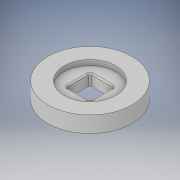
# Autodesk Inventor part: gear_collar_small
Saved by Autodesk Inventor 2019.3 (Build 233278000, 278)
## iProperties
Created: 2019-01-25
Part Number: gear_collar_small
Material: Generic
Document SubType Name: Modeling
Designer: Varga Daniel
Density: 1 g/cm^3
Appearance: Default
Author: Varga Daniel
Autodesk Inventor part; units mm, degrees
ref_plane "YZ Plane" through (0, 0, 0) normal (1, 0, 0) x (0, 1, 0)
ref_plane "XZ Plane" through (0, 0, 0) normal (0, 1, 0) x (-1, 0, 0)
ref_plane "XY Plane" through (0, 0, 0) normal (0, 0, 1) x (1, 0, 0)
derived "Base_part.ipt"
sketch "Axle_hole_sketch" plane through (0, 0, 0) normal (0, 1, 0) x (-1, 0, 0)
  line L0 (-14.3207, 2.4447) -> (-17.4707, 2.4447)
  line L1 (-17.7707, 2.7447) -> (-17.7707, 5.8947)
  line L2 (-17.4707, 6.1947) -> (-14.3207, 6.1947)
  line L3 (-14.0207, 5.8947) -> (-14.0207, 2.7447)
  line L4 (-14.0207, 2.4447) -> (-17.7707, 6.1947) construction
  line L5 (-17.7707, 2.4447) -> (-14.0207, 6.1947) construction
  arc A0 (-14.3207, 2.4447) -> (-14.0207, 2.7447) centre (-14.3207, 2.7447) ccw
  arc A1 (-17.7707, 2.7447) -> (-17.4707, 2.4447) centre (-17.4707, 2.7447) ccw
  arc A2 (-17.4707, 6.1947) -> (-17.7707, 5.8947) centre (-17.4707, 5.8947) ccw
  arc A3 (-14.0207, 5.8947) -> (-14.3207, 6.1947) centre (-14.3207, 5.8947) ccw
  point P0 (0, 0)
  point P1 (-15.8957, 4.3197)
sketch "Sketch1" plane through (0, 0, 0) normal (0, 1, 0) x (-1, 0, 0)
  circle A0 centre (0, 0) radius 6.5
  dimension "d2" = 13
  constraints: 1 centre point, 1 coincident
  measures "d2" diameter of A0
extrude "Extrusion1" add sketch "Sketch1" along normal blind 2.5
sketch "Sketch2" plane through (0, 2.5, 0) normal (0, 1, 0) x (1, 0, 0)
  line L0 (-1.575, -1.875) -> (1.575, -1.875)
  line L1 (1.875, -1.575) -> (1.875, 1.575)
  line L2 (1.575, 1.875) -> (-1.575, 1.875)
  line L3 (-1.875, 1.575) -> (-1.875, -1.575)
  line L4 (-1.875, -1.875) -> (1.875, 1.875) construction
  line L5 (1.875, -1.875) -> (-1.875, 1.875) construction
  arc A0 (-1.575, 1.875) -> (-1.875, 1.575) centre (-1.575, 1.575) ccw
  arc A1 (-1.875, -1.575) -> (-1.575, -1.875) centre (-1.575, -1.575) ccw
  arc A2 (1.575, -1.875) -> (1.875, -1.575) centre (1.575, -1.575) ccw
  arc A3 (1.875, 1.575) -> (1.575, 1.875) centre (1.575, 1.575) ccw
  line L6 (14.3207, -2.4447) -> (17.4707, -2.4447) construction
  line L7 (14.0207, -5.8947) -> (14.0207, -2.7447) construction
  arc A4 (14.3207, -2.4447) -> (14.0207, -2.7447) centre (14.3207, -2.7447) ccw construction
  line L8 (17.7707, -2.7447) -> (17.7707, -5.8947) construction
  arc A5 (17.7707, -2.7447) -> (17.4707, -2.4447) centre (17.4707, -2.7447) ccw construction
  arc A6 (17.4707, -6.1947) -> (17.7707, -5.8947) centre (17.4707, -5.8947) ccw construction
  line L9 (17.4707, -6.1947) -> (14.3207, -6.1947) construction
  arc A7 (14.0207, -5.8947) -> (14.3207, -6.1947) centre (14.3207, -5.8947) ccw construction
  point P0 (0, 0)
  dimension "d5" = 3.75
  dimension "d6" = 3.75
  dimension "d7" = 0.3
  dimension "d15" = 3.75
  dimension "d16" = 0.3
  constraints: 12 end point, 8 point on circle, 8 point on line, 8 tangent, 4 centre point, 3 equal radius, 2 midpoint, 2 parallel, 1 horizontal, 1 perpendicular
  measures "d5" distance of L5.end L4.end
  measures "d6" distance between parallel lines of L0 L2
  measures "d7" radius of A0
  measures "d15" distance between parallel lines of L7 L8
  measures "d16" radius of A5
extrude "Extrusion2" cut sketch "Sketch2" against normal through all
sketch "Sketch3" plane through (0, 2.5, 0) normal (0, 1, 0) x (1, 0, 0)
  circle A0 centre (0, 0) radius 4
  dimension "d10" = 8
  constraints: 1 centre point, 1 coincident
  measures "d10" diameter of A0
extrude "Extrusion3" cut sketch "Sketch3" against normal blind 0.8
fillet "Fillet1" radius 0.2 8 edges at (-1.7871, 1.7, 1.7871) (0, 1.7, 1.875) (1.7871, 1.7, 1.7871) (1.875, 1.7, 0) (1.7871, 1.7, -1.7871) (0, 1.7, -1.875) (-1.7871, 1.7, -1.7871) (-1.875, 1.7, 0)
equation "\"d5\" = d15"
equation "\"d6\" = d5"
equation "\"d7\" = d16"
body "Solid1"
